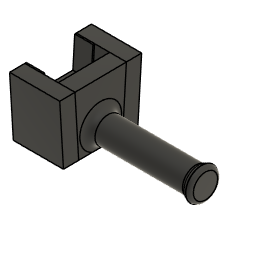
a6147cae-77b5-46f0-ad01-8fbcf3883dca (Autodesk Fusion 360 design; units mm, degrees)
Autodesk Fusion 360 part; units mm, degrees
sketch "Esboço1" plane through (0, 0, 0.7) normal (0, 0, 1) x (-0.01044, 0.999946, 0)
  line L0 (-3.0443, -6.2687) -> (-1.7592, 11.6516)
  arc A0 (-8.9454, 11.7266) -> (-1.7592, 11.6516) centre (-5.35, 11.9091) ccw
  line L1 (-8.9454, 11.7266) -> (-8.0347, -6.2166)
  arc A1 (-8.0347, -6.2166) -> (-3.0443, -6.2687) centre (-5.5379, -6.0899) ccw
  line L2 (-2.8098, -2.9991) -> (-8.198, -2.9991)
  line L3 (-8.604, 5.0009) -> (-2.2362, 5.0009)
  line L4 (-2.6093, -2.9991) -> (-2.0356, 5.0009)
  line L5 (-8.8043, 5.0009) -> (-8.3983, -2.9991)
  line L6 (-0.762, -5.1991) -> (-0.0305, 5.0009)
  line L7 (-10.8069, 5.0009) -> (-10.4008, -2.9991)
  line L8 (-2.8098, -2.9991) -> (-0.6042, -2.9991)
  line L9 (-8.198, -2.9991) -> (-10.4008, -2.9991)
  line L10 (-2.2362, 5.0009) -> (-0.0305, 5.0009)
  line L11 (-8.604, 5.0009) -> (-10.8069, 5.0009)
  line L12 (-5.5039, -2.9991) -> (-5.4201, 5.0009) construction
  circle A2 centre (-5.4777, -0.4991) radius 1.75
  line L13 (-2.3225, 1.0009) -> (-8.6013, 1.0009)
  dimension "d557" = 8
  dimension "d572" = 3.5
  dimension "d573" = 2.5
  dimension "d574" = 4
  constraint coincident L0 L2.start
  constraint coincident L1 L2.end
  constraint horizontal L2
  constraint coincident L1 L3.start
  constraint coincident L0 L3.end
  constraint horizontal L3
  constraint coincident L6 L8.end
  constraint parallel L2 L8
  constraint parallel L8 L9
  constraint parallel L3 L10
  constraint parallel L3 L11
  constraint coincident L11 L5.start
  constraint coincident L10 L4.end
  constraint coincident L8 L4.start
  constraint coincident L9 L5.end
  constraint midpoint L2 L12.start
  constraint midpoint L3 L12.end
  constraint coincident L12 A2.centre
  constraint coincident L4 L13.start
  constraint coincident L5 L13.end
  constraint horizontal L13
  measures "d557" distance of L2 L3
  measures "d572" diameter of A2
  measures "d573" distance of L2 A2.centre
  measures "d574" distance of L3 L13
extrude "Extrusão1" add sketch "Esboço1" along normal blind 2.2 contours L0 L1 L2 A2 L13 | L0 L4 L8 L13 | L0 L1 L3 A2 L13 | L0 L4 L10 L13 | L1 L5 L9 L13 | A2 L13 | A2 L13 | L1 L5 L11 L13 makes body 1
extrude "Extrusão2" add sketch "Esboço1" along normal blind -4.4 and the other way blind -2.2 separate body contours L4 L6 L8 L10 | L5 L7 L9 L11 makes body 2 at (0.3577, -2.4145, 0.7) makes body 3 at (-2.2227, -10.6953, 0.7)
extrude "Extrusão3" add sketch "Esboço1" along normal blind -2 and the other way blind 4.4 separate body contours L0 L1 L2 A2 L13 | L0 L4 L8 L13 | L0 L4 L10 L13 | L1 L5 L9 L13 | A2 L13 | L1 L5 L11 L13 picked at (-5.5543, -0.1525) makes body 4
extrude "Extrusão4" add sketch "Esboço1" along normal blind 16 contours A2 L13 | A2 L13 bodies 1
sketch "Esboço2" plane through (0, 0, 16.7) normal (0, 0, 1) x (1, 0, 0)
  circle A0 centre (0.5563, -5.4722) radius 1.75
  circle A1 centre (0.5563, -5.4722) radius 2.1
  dimension "d577" = 4.2
  constraint concentric A0 A1
  measures "d577" diameter of A1
extrude "Extrusão5" add sketch "Esboço2" against normal blind 1 bodies 1
fillet "Arredondamento1" radius 0.5 3 edges at (-1.4016, -4.7128, 15.7) (-0.0595, -7.1103, 15.7) (-1.4016, -6.2316, 16.7) on bodies 1
fillet "Arredondamento2" radius 1 1 edges at (-0.0595, -7.1103, 2.9) on bodies 1
move_body "Mover1" bodies 2 3 4 1 to x (0, 0, -1) y (0, 1, 0) z (1, 0, 0) at (-3.887, 0, 1.913)
